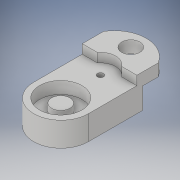
# Autodesk Inventor part: top hand base with 2 gears
Saved by Autodesk Inventor 2018 (Build 220112000, 112)
## iProperties
Created: 2017-10-01
Part Number: top hand base with 2 gears
Material: Generic
Document SubType Name: Modeling
Designer: Martin
Density: 1 g/cm^3
Appearance: Default
Author: Martin
Autodesk Inventor part; units mm, degrees
ref_plane "YZ Plane" through (0, 0, 0) normal (1, 0, 0) x (0, 1, 0)
ref_plane "XZ Plane" through (0, 0, 0) normal (0, 1, 0) x (-1, 0, 0)
ref_plane "XY Plane" through (0, 0, 0) normal (0, 0, 1) x (1, 0, 0)
sketch "Sketch1" plane through (0, 0, 0) normal (0, 1, 0) x (-1, 0, 0)
  line L0 (18, 0) -> (18, -30)
  line L1 (18, -30) -> (0, -30)
  line L2 (0, -30) -> (0, 0)
  arc A0 (18, 0) -> (0, 0) centre (9, 0) ccw
  circle A1 centre (9, -23) radius 1
  circle A2 centre (9, -13) radius 1
  dimension "d6" = 2
  dimension "d8" = 2
  constraints: 6 end point, 3 centre point, 2 point on circle, 1 parallel, 1 tangent
  measures "d6" diameter of A1
  measures "d8" diameter of A2
extrude "Extrusion1" add sketch "Sketch1" along normal blind 8
sketch "Sketch2" plane through (0, 8, 0) normal (0, 1, 0) x (1, 0, 0)
  circle A0 centre (-9.1017, 0) radius 3
  circle A1 centre (-9.1017, 0) radius 7
  point P0 (0, 0)
  dimension "d11" = 6
  dimension "d12" = 14
  constraints: 2 centre point, 1 coincident
  measures "d11" diameter of A0
  measures "d12" diameter of A1
extrude "Extrusion2" cut sketch "Sketch2" against normal blind 4
sketch "Sketch3" plane through (-9.1017, 8, 0) normal (0, 1, 0) x (1, 0, 0)
  circle A0 centre (0, 0) radius 3
  point P0 (9.1017, 0)
  constraints: 1 centre point
extrude "Extrusion3" cut sketch "Sketch3" against normal blind 1.5
sketch "Sketch4" plane through (0, 8, 0) normal (0, 1, 0) x (1, 0, 0)
  line L0 (0, 23) -> (0, 16)
  line L1 (0, 16) -> (-18, 16)
  line L2 (-18, 16) -> (-18, 23)
  circle A0 centre (-9, 23) radius 3
  arc A1 (0, 23) -> (-18, 23) centre (-9, 17.5917) ccw
  point P0 (0, 0)
  dimension "d17" = 18
  constraints: 6 end point, 2 centre point, 2 point on circle, 1 parallel
  measures "d17" distance of L0.end L1.end
extrude "Extrusion4" add sketch "Sketch4" along normal blind 3
sketch "Sketch6" plane through (0, 0, 0) normal (0, -1, 0) x (1, 0, 0)
  line L0 (0, 0) -> (0, -30) projected
  line L1 (-18, -30) -> (-18, 0) projected
  line L2 (0, -30) -> (-18, -30)
  line L3 (-18, -30) -> (-18, -18)
  line L4 (-18, -18) -> (0, -18)
  line L5 (0, -18) -> (0, -30)
  dimension "d23" = 12
  constraints: 8 end point, 2 parallel, 1 horizontal, 1 perpendicular, 1 point on line
  measures "d23" distance of L2.end L3.end
extrude "Extrusion5" cut sketch "Sketch6" against normal blind 7
sketch "Sketch7" plane through (0, 8, 0) normal (0, 1, 0) x (1, 0, 0)
  circle A0 centre (-9, 23) radius 3
  point P0 (0, 0)
  point P1 (-18, 23)
  point P2 (0, 30)
  point P3 (-6, 23)
  point P4 (-12, 23)
  constraints: 2 point on circle, 1 centre point, 1 coincident
extrude "Extrusion6" cut sketch "Sketch7" against normal through all
sketch "Sketch8" plane through (0, 8, 0) normal (0, 1, 0) x (1, 0, 0)
  line L0 (-18, 30) -> (-18, 23) projected
  arc A0 (0, 23) -> (-18, 23) centre (-9, 17.5917) ccw
  line L1 (0, 30) -> (-18, 30) projected
  line L2 (3.2096, 23) -> (3.2096, 32.8991)
  line L3 (3.2096, 32.8991) -> (-22.1602, 32.8991)
  line L4 (-22.1602, 32.8991) -> (-22.1602, 23)
  line L5 (-22.1602, 23) -> (-18, 23)
  line L6 (0, 23) -> (3.2096, 23)
  point P0 (0, 0)
  constraints: 10 end point, 3 parallel, 2 horizontal, 2 perpendicular, 2 point on circle, 1 centre point
extrude "Extrusion7" cut sketch "Sketch8" against normal blind 7
sketch "Sketch11" plane through (0, 11, 0) normal (0, 1, 0) x (1, 0, 0)
  circle A0 centre (-9, 13) radius 1 projected
  circle A1 centre (-9, 13) radius 5
  point P0 (0, 0)
  dimension "d34" = 10
  constraints: 1 centre point, 1 coincident
  measures "d34" diameter of A1
extrude "Extrusion9" cut sketch "Sketch11" against normal blind 3
body "Solid1"
